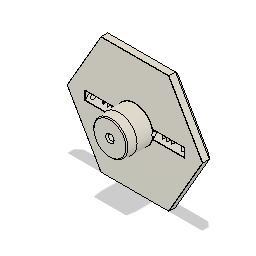
Madla skříně v pracovně II v6 (Autodesk Fusion 360 design; units mm, degrees)
Autodesk Fusion 360 part; units mm, degrees
sketch "Sketch1" plane through (0, 0, 0) normal (0, 0, 1) x (1, 0, 0)
  line L0 (15, -25.9808) -> (30, 0)
  line L1 (30, 0) -> (15, 25.9808)
  line L2 (15, 25.9808) -> (-15, 25.9808)
  line L3 (-15, 25.9808) -> (-30, 0)
  line L4 (-30, 0) -> (-15, -25.9808)
  line L5 (-15, -25.9808) -> (15, -25.9808)
  circle A0 centre (0, 0) radius 8
  circle A1 centre (0, 0) radius 20 construction
  circle A2 centre (0, 0) radius 1.25
  point P0 (20, 0)
  point P1 (-20, 0)
  dimension "d1" = 30
  dimension "d2" = 16
  dimension "d3" = 40
  dimension "d4" = 2.5
  constraint coincident A0.centre A1.centre
  constraint horizontal L0.end A0.centre
  constraint coincident A1 P0
  constraint coincident A1 P1
  constraint horizontal A0.centre P1
  constraint horizontal A0.centre P0
  measures "d1" distance of L0.start A0.centre
  measures "d2" diameter of A0
  measures "d3" diameter of A1
  measures "d4" diameter of A2
extrude "Extrude1" add sketch "Sketch1" against normal blind 5 contours L0 L1 L2 L3 L4 L5 | A0 | A2
extrude "Extrude2" add sketch "Sketch1" along normal blind 11 contours A0
sketch "Sketch2" plane through (0, 0, 0) normal (1, 0, 0) x (0, 0, -1)
  line L0 (0, 0) -> (0, 25.9808)
  line L1 (0, -25.9808) -> (0, 0)
  line L2 (0, 0) -> (5, 0)
  circle A0 centre (0.5, 0) radius 1
  line L3 (0, -1.9142) -> (1.9142, 0)
  line L4 (1.9142, 0) -> (0, 1.9142)
  dimension "d9" = 2
  dimension "d10" = 0.5
  dimension "d11" = 90
  constraint horizontal A0.centre L0.start
  constraint coincident L1 L3.start
  constraint coincident L2 L3.end
  constraint coincident L0 L4.end
  constraint tangent A0 L3
  constraint tangent A0 L4
  measures "d9" diameter of A0
  measures "d10" distance of A0.centre L0.start
  measures "d11" angle of L3 L4
extrude "Extrude3" cut sketch "Sketch2" along normal blind 7 from surface at 1 contours L0 L1 A0 | L1 L2 A0 | L0 L2 A0
extrude "Extrude4" cut sketch "Sketch2" along normal blind 14 from surface at 8 contours L1 L2 A0 | L0 L2 A0 | L0 A0 L4 | L1 A0 L3 | L2 A0 L4 | L2 A0 L3
hole "Hole1" at (20, 0, 0) direction (0, 0, -1) diameter 2 end through all
sketch "Sketch3" plane through (0, 0, 0) normal (0, 1, 0) x (1, 0, 0)
  arc A0 (19, 1.9142) -> (21, 1.9142) centre (20, 1.9142) ccw
  line L0 (21, 1.9142) -> (22, 1.9142)
  line L1 (22, 1.9142) -> (22, 0)
  line L2 (22, 0) -> (8, 0)
  line L3 (8, 0) -> (8, 1.2071)
  line L4 (8, 1.2071) -> (8, 1.9142)
  line L5 (8, 1.9142) -> (19, 1.9142)
  line L6 (11, 1.9142) -> (11.1, 1.1142)
  line L7 (11.1, 1.1142) -> (12.2, 1.9142)
  line L8 (13, 1.9142) -> (13.1, 1.1142)
  line L9 (13.1, 1.1142) -> (14.2, 1.9142)
  line L10 (15, 1.9142) -> (15.1, 1.1142)
  line L11 (15.1, 1.1142) -> (16.2, 1.9142)
  dimension "d21" = 1.2
  dimension "d22" = 0.8
  dimension "d25" = 0.1
  dimension "d28" = 2
  dimension "d29" = 0
  dimension "d30" = 3
  constraint horizontal L6.start L7.end
  constraint coincident L5 L6.start
  measures "d21" distance of L6.start L7.end
  measures "d22" vertical distance of L6.end L7.end
  measures "d25" horizontal distance of L6.start L6.end
  measures "d30" distance of L4.end L6.start
extrude "Extrude5" add sketch "Sketch3" along normal mid plane 2 contours L5 L10 L11 | L5 L8 L9 | L5 L6 L7
mirror "Mirror1" about plane through (0, 0, 0) normal (1, 0, 0) of "Extrude3", "Extrude4", "Hole1", "Extrude5"
chamfer "Chamfer1" distance 2 angle 45 6 edges at (0, -25.9808, -5) (22.5, -12.9904, -5) (22.5, 12.9904, -5) (0, 25.9808, -5) (-22.5, 12.9904, -5) (-22.5, -12.9904, -5)
chamfer "Chamfer2" distance 0.1 angle 45 1 faces at (0, -19.9872, 0)
chamfer "Chamfer3" distance 0.5 distance2 4 1 edges at (-7.4586, -2.8929, 11) measured on face at (5.7156, -0.4595, 11)
chamfer "Chamfer4" distance 0.4 angle 45 1 edges at (-6.9925, 2.7121, 11)
chamfer "Chamfer5" distance 0.4 angle 45 2 edges at (-19.0677, -0.3616, -5) (19.0677, -0.3616, -5)
chamfer "Chamfer6" distance 0.6 angle 45 1 edges at (-1.1654, 0.452, 11)
named bodies: "Madlo II"
